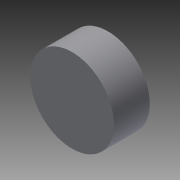
# Autodesk Inventor part: connectors
Saved by Autodesk Inventor 2015 (Build 190159000, 159)
## iProperties
Created: 2015-07-03
Part Number: connectors
Material: Generic
Document SubType Name: Modeling
Designer: Sudhar
Density: 1 g/cm^3
Appearance: Default
Author: Sudhar
Autodesk Inventor part; units mm, degrees
ref_plane "YZ Plane" through (0, 0, 0) normal (1, 0, 0) x (0, 1, 0)
ref_plane "XZ Plane" through (0, 0, 0) normal (0, 1, 0) x (-1, 0, 0)
ref_plane "XY Plane" through (0, 0, 0) normal (0, 0, 1) x (1, 0, 0)
sketch "Sketch1" plane through (0, 0, 0) normal (0, 0, 1) x (1, 0, 0)
  circle A0 centre (2.6037, 2.6595) radius 8.89
  dimension "d0" = 17.78
  constraints: 1 centre point
  measures "d0" diameter of A0
extrude "Extrusion1" add sketch "Sketch1" along normal blind 7.62
sketch "Sketch2" plane through (2.6037, 2.6595, 0) normal (0, 0, -1) x (-1, 0, 0)
  circle A0 centre (0, 0) radius 3.81
  dimension "d3" = 7.62
  constraints: 1 centre point
  measures "d3" diameter of A0
extrude "Extrusion2" cut sketch "Sketch2" against normal blind 1.27
body "Solid1"
